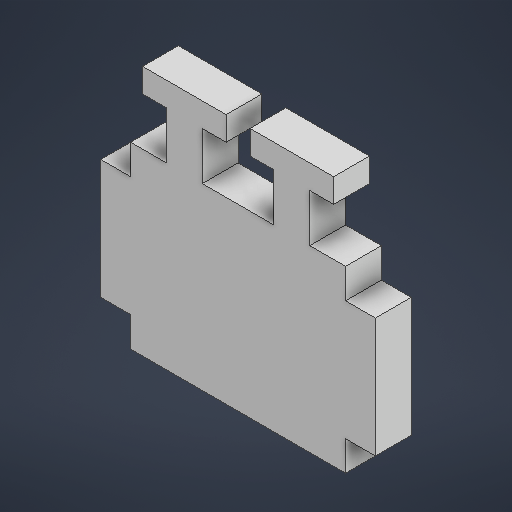
# Autodesk Inventor part: Spring_holder2
Saved by Autodesk Inventor 2027 (Build 310192000, 192)
## iProperties
Created: 2026-05-09
Part Number: Spring_holder2
Material: Generic
Document SubType Name: Modeling
Designer: alexy
Density: 1 g/cm^3
Appearance: Default
Author: alexy
Autodesk Inventor part; units mm, degrees
ref_plane "YZ Plane" through (0, 0, 0) normal (1, 0, 0) x (0, 1, 0)
ref_plane "XZ Plane" through (0, 0, 0) normal (0, 1, 0) x (-1, 0, 0)
ref_plane "XY Plane" through (0, 0, 0) normal (0, 0, 1) x (1, 0, 0)
sketch "Sketch1" plane through (0, 0, 0) normal (0, 0, 1) x (1, 0, 0)
  line L0 (0, 0) -> (18, 0)
  line L1 (18, 0) -> (18, 15)
  line L2 (18, 15) -> (0, 15)
  line L3 (0, 15) -> (0, 0)
  line L4 (20.5, 12.5) -> (18, 12.5)
  line L5 (18, 12.5) -> (18, 2.5)
  line L6 (18, 2.5) -> (20.5, 2.5)
  line L7 (20.5, 2.5) -> (20.5, 12.5)
  line L8 (20.5, 12.5) -> (18, 2.5) construction
  line L9 (18, 12.5) -> (20.5, 2.5) construction
  line L10 (-2.5, 12.5) -> (0, 12.5)
  line L11 (0, 12.5) -> (0, 2.5)
  line L12 (0, 2.5) -> (-2.5, 2.5)
  line L13 (-2.5, 2.5) -> (-2.5, 12.5)
  line L14 (-2.5, 12.5) -> (0, 2.5) construction
  line L15 (0, 12.5) -> (-2.5, 2.5) construction
  line L16 (3, 15) -> (3, 19)
  line L17 (3, 19) -> (1, 19)
  line L18 (1, 19) -> (1, 21)
  line L19 (1, 21) -> (8, 21)
  line L20 (8, 21) -> (8, 19)
  line L21 (8, 19) -> (6, 19)
  line L22 (6, 19) -> (6, 15)
  line L23 (12, 15) -> (12, 19)
  line L24 (12, 19) -> (10, 19)
  line L25 (10, 19) -> (10, 21)
  line L26 (10, 21) -> (17, 21)
  line L27 (17, 21) -> (17, 19)
  line L28 (17, 19) -> (15, 19)
  line L29 (15, 19) -> (19.0944, 19)
  line L30 (15, 19) -> (15, 15)
  point P0 (19.25, 7.5)
  point P1 (-1.25, 7.5)
  point P2 (18, 7.5)
  point P3 (0, 7.5)
  point P4 (0, 12.5)
  dimension "d0" = 18
  dimension "d1" = 15
  dimension "d2" = 2.5
  dimension "d3" = 2.5
  dimension "d4" = 10
  dimension "d5" = 4
  dimension "d6" = 2
  dimension "d7" = 2
  dimension "d8" = 7
  dimension "d9" = 2
  dimension "d10" = 2
  dimension "d11" = 3
  dimension "d21" = 4
  dimension "d22" = 2
  dimension "d23" = 2
  dimension "d24" = 7
  dimension "d25" = 2
  dimension "d26" = 2
  dimension "d27" = 3
  constraints: 62 end point, 10 perpendicular, 10 point on line, 6 midpoint, 6 parallel, 4 horizontal, 3 horizontal alignment, 3 vertical
  measures "d0" distance of L2.end L1.end
  measures "d1" distance of L0.end L1.end
  measures "d2" distance of L5.end L6.end
  measures "d3" distance of L11.end L12.end
  measures "d4" distance of L12.end L10.start
  measures "d5" distance of L16.start L16.end
  measures "d6" distance of L16.end L17.end
  measures "d7" distance of L17.end L18.end
  measures "d8" distance of L18.end L19.end
  measures "d9" distance of L19.end L20.end
  measures "d10" distance of L20.end L21.end
  measures "d11" distance from line of L2.end L16
  measures "d21" distance of L23.start L23.end
  measures "d22" distance of L23.end L24.end
  measures "d23" distance of L24.end L25.end
  measures "d24" distance of L25.end L27.start
  measures "d25" distance of L27.start L28.start
  measures "d26" distance of L28.start L29.start
  measures "d27" distance of L1.end L30.end
extrude "Extrusion1" add sketch "Sketch1" along normal blind 3
body "Solid1"
